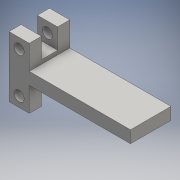
# Autodesk Inventor part: promo_hold
Saved by Autodesk Inventor 2016 (Build 200138000, 138)
## iProperties
Created: 2016-05-11
Part Number: promo_hold
Material: 一般
Document SubType Name: Modeling
Designer: 宏太
Density: 1 g/cm^3
Appearance: 既定
Mass: 1.20968 g
Surface Area: 13.3781 cm^2
Volume: 1.20968 cm^3
Author: 宏太
Autodesk Inventor part; units mm, degrees
ref_plane "YZ Plane" through (0, 0, 0) normal (1, 0, 0) x (0, 1, 0)
ref_plane "XZ Plane" through (0, 0, 0) normal (0, 1, 0) x (-1, 0, 0)
ref_plane "XY Plane" through (0, 0, 0) normal (0, 0, 1) x (1, 0, 0)
sketch "スケッチ1" plane through (0, 0, 0) normal (0, 1, 0) x (-1, 0, 0)
  line L0 (-15, -7.5) -> (15, -7.5)
  line L1 (15, -7.5) -> (15, 7.5)
  line L2 (15, 7.5) -> (-15, 7.5)
  line L3 (-15, 7.5) -> (-15, -7.5)
  line L4 (-15, -7.5) -> (15, 7.5) construction
  line L5 (15, -7.5) -> (-15, 7.5) construction
  point P0 (0, 0)
  dimension "d0" = 30
  dimension "d1" = 15
  constraints: 12 end point, 2 midpoint, 2 parallel, 1 horizontal, 1 perpendicular
  measures "d0" distance of L2.end L1.end
  measures "d1" distance of L1.end L0.end
extrude "押し出し1" add sketch "スケッチ1" along normal mid plane 10
sketch "スケッチ2" plane through (0, 0, 0) normal (0, 1, 0) x (-1, 0, 0)
  line L0 (15, 7.5) -> (-15, 7.5) projected
  line L1 (10, 7.5) -> (-15, 7.5)
  line L2 (-15, 7.5) -> (-15, 1.5)
  line L3 (-15, 1.5) -> (10, 1.5)
  line L4 (10, 1.5) -> (10, 7.5)
  point P0 (0, 0)
  dimension "d4" = 25
  dimension "d5" = 6
  dimension "d6" = 5
  constraints: 8 end point, 2 parallel, 1 horizontal, 1 perpendicular, 1 point on line
  measures "d4" distance of L3.end L2.end
  measures "d5" distance of L2.end L1.end
  measures "d6" distance from line of L0.start L4
extrude "押し出し2" cut sketch "スケッチ2" along normal mid plane 10
sketch "スケッチ3" plane through (0, 0, 0) normal (0, 1, 0) x (-1, 0, 0)
  line L0 (15, -7.5) -> (-15, -7.5) projected
  line L1 (-15, -7.5) -> (10, -7.5)
  line L2 (10, -7.5) -> (10, -1.5)
  line L3 (10, -1.5) -> (-15, -1.5)
  line L4 (-15, -1.5) -> (-15, -7.5)
  point P0 (0, 0)
  dimension "d9" = 25
  dimension "d10" = 6
  constraints: 8 end point, 2 parallel, 1 horizontal, 1 perpendicular
  measures "d9" distance of L3.end L2.end
  measures "d10" distance of L2.end L1.end
extrude "押し出し3" cut sketch "スケッチ3" along normal mid plane 10
sketch "スケッチ4" plane through (0, 0, 0) normal (1, 0, 0) x (0, 1, 0)
  line L0 (2, 7.5) -> (-2, 7.5)
  line L1 (-2, 7.5) -> (-2, 2.5)
  line L2 (-2, 2.5) -> (2, 2.5)
  line L3 (2, 2.5) -> (2, 7.5)
  point P0 (0, 0)
  dimension "d13" = 4
  dimension "d14" = 5
  dimension "d15" = 2
  dimension "d16" = 7.5
  constraints: 8 end point, 2 parallel, 1 horizontal, 1 perpendicular
  measures "d13" distance of L2.end L1.end
  measures "d14" distance of L1.end L0.end
  measures "d15" distance from line of point (0, 0) L3
  measures "d16" distance from line of point (0, 0) L0
extrude "押し出し4" cut sketch "スケッチ4" against normal blind 15
sketch "スケッチ6" plane through (0, 5, 0) normal (0, 1, 0) x (1, 0, 0)
  circle A0 centre (-12.5, -5) radius 1.25
  line L0 (-15, -7.5) -> (-10, -7.5) projected
  point P0 (0, 0)
  dimension "d23" = 2.5
  dimension "d24" = 2.5
  constraints: 1 centre point
  measures "d23" diameter of A0
  measures "d24" distance from line of L0 A0.centre
extrude "押し出し5" cut sketch "スケッチ6" against normal blind 15
sketch "スケッチ7" plane through (0, 5, 0) normal (0, 1, 0) x (1, 0, 0)
  circle A0 centre (-12.5, 5) radius 1.25
  line L0 (-10, 7.5) -> (-15, 7.5) projected
  line L1 (-15, 7.5) -> (-15, -7.5) projected
  point P0 (0, 0)
  dimension "d27" = 2.5
  dimension "d28" = 2.5
  constraints: 1 centre point
  measures "d27" diameter of A0
  measures "d28" distance from line of L0 A0.centre
extrude "押し出し6" cut sketch "スケッチ7" against normal blind 15
sketch "スケッチ8" plane through (-10, -5, -1.5) normal (1, 0, 0) x (0, 0, -1)
  line L0 (1, 7) -> (6, 7)
  line L1 (6, 7) -> (6, 3)
  line L2 (6, 3) -> (1, 3)
  line L3 (1, 3) -> (1, 7)
  point P0 (-1.5, 5)
  dimension "d32" = 5
  dimension "d33" = 4
  dimension "d34" = 7.5
  dimension "d35" = 2
  constraints: 8 end point, 2 parallel, 1 horizontal, 1 perpendicular
  measures "d32" distance of L1.end L2.end
  measures "d33" distance of L0.end L1.end
  measures "d34" distance from line of point (-1.5, 5) L1
  measures "d35" distance from line of point (-1.5, 5) L0
extrude "押し出し7" cut sketch "スケッチ8" against normal blind 15
